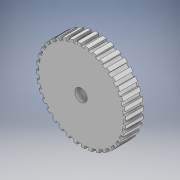
# Autodesk Inventor part: IPC BRT Knob
Saved by Autodesk Inventor 2022 (Build 260153000, 153)
## iProperties
Created: 2022-01-01
Part Number: IPC BRT Knob
Material: Generic
Document SubType Name: Modeling
Designer: solor
Density: 1 g/cm^3
Appearance: Default
Author: solor
Autodesk Inventor part; units mm, degrees
ref_plane "YZ Plane" through (0, 0, 0) normal (1, 0, 0) x (0, 1, 0)
ref_plane "XZ Plane" through (0, 0, 0) normal (0, 1, 0) x (-1, 0, 0)
sketch "Sketch1" plane through (0, 0, 0) normal (0, 0, 1) x (1, 0, 0)
  arc A0 (21.6935, 0) -> (21.6109, 1.8907) centre (0, 0) ccw
  arc A1 (20.422, 1.7867) -> (20.1886, 3.5598) centre (0, 0) ccw
  line L0 (20.422, 1.7867) -> (21.6109, 1.8907)
  line L1 (20.1886, 3.5598) -> (21.3639, 3.767)
  arc A2 (21.3639, 3.767) -> (20.9543, 5.6147) centre (0, 0) ccw
  arc A3 (19.8015, 5.3058) -> (19.2637, 7.0114) centre (0, 0) ccw
  line L2 (19.8015, 5.3058) -> (20.9543, 5.6147)
  line L3 (19.2637, 7.0114) -> (20.3852, 7.4196)
  arc A4 (20.3852, 7.4196) -> (19.661, 9.1681) centre (0, 0) ccw
  arc A5 (18.5793, 8.6637) -> (17.7535, 10.25) centre (0, 0) ccw
  line L4 (18.5793, 8.6637) -> (19.661, 9.1681)
  line L5 (17.7535, 10.25) -> (18.7871, 10.8468)
  arc A6 (18.7871, 10.8467) -> (17.7703, 12.4429) centre (0, 0) ccw
  arc A7 (16.7926, 11.7583) -> (15.7039, 13.1771) centre (0, 0) ccw
  line L6 (16.7926, 11.7583) -> (17.7703, 12.4429)
  line L7 (15.7039, 13.1771) -> (16.6182, 13.9443)
  arc A8 (16.6182, 13.9443) -> (15.3396, 15.3396) centre (0, 0) ccw
  arc A9 (14.4957, 14.4957) -> (13.1771, 15.7039) centre (0, 0) ccw
  line L8 (14.4957, 14.4957) -> (15.3396, 15.3396)
  line L9 (13.1771, 15.7039) -> (13.9443, 16.6182)
  arc A10 (13.9443, 16.6182) -> (12.4429, 17.7703) centre (0, 0) ccw
  arc A11 (11.7583, 16.7926) -> (10.25, 17.7535) centre (0, 0) ccw
  line L10 (11.7583, 16.7926) -> (12.4429, 17.7703)
  line L11 (10.25, 17.7535) -> (10.8468, 18.7871)
  arc A12 (10.8468, 18.7871) -> (9.1681, 19.661) centre (0, 0) ccw
  arc A13 (8.6637, 18.5793) -> (7.0114, 19.2637) centre (0, 0) ccw
  line L12 (8.6637, 18.5793) -> (9.1681, 19.661)
  line L13 (7.0114, 19.2637) -> (7.4196, 20.3852)
  arc A14 (7.4196, 20.3852) -> (5.6147, 20.9543) centre (0, 0) ccw
  arc A15 (5.3058, 19.8015) -> (3.5598, 20.1886) centre (0, 0) ccw
  line L14 (5.3058, 19.8015) -> (5.6147, 20.9543)
  line L15 (3.5598, 20.1886) -> (3.767, 21.3639)
  arc A16 (3.767, 21.3639) -> (1.8907, 21.6109) centre (0, 0) ccw
  arc A17 (1.7867, 20.422) -> (0, 20.5) centre (0, 0) ccw
  line L16 (1.7867, 20.422) -> (1.8907, 21.6109)
  line L17 (0, 20.5) -> (0, 21.6935)
  arc A18 (0, 21.6935) -> (-1.8907, 21.6109) centre (0, 0) ccw
  arc A19 (-1.7867, 20.422) -> (-3.5598, 20.1886) centre (0, 0) ccw
  line L18 (-1.7867, 20.422) -> (-1.8907, 21.6109)
  line L19 (-3.5598, 20.1886) -> (-3.767, 21.3639)
  arc A20 (-3.767, 21.3639) -> (-5.6147, 20.9543) centre (0, 0) ccw
  arc A21 (-5.3058, 19.8015) -> (-7.0114, 19.2637) centre (0, 0) ccw
  line L20 (-5.3058, 19.8015) -> (-5.6147, 20.9543)
  line L21 (-7.0114, 19.2637) -> (-7.4196, 20.3852)
  arc A22 (-7.4196, 20.3852) -> (-9.1681, 19.661) centre (0, 0) ccw
  arc A23 (-8.6637, 18.5793) -> (-10.25, 17.7535) centre (0, 0) ccw
  line L22 (-8.6637, 18.5793) -> (-9.1681, 19.661)
  line L23 (-10.25, 17.7535) -> (-10.8468, 18.7871)
  arc A24 (-10.8467, 18.7871) -> (-12.4429, 17.7703) centre (0, 0) ccw
  arc A25 (-11.7583, 16.7926) -> (-13.1771, 15.7039) centre (0, 0) ccw
  line L24 (-11.7583, 16.7926) -> (-12.4429, 17.7703)
  line L25 (-13.1771, 15.7039) -> (-13.9443, 16.6182)
  arc A26 (-13.9443, 16.6182) -> (-15.3396, 15.3396) centre (0, 0) ccw
  arc A27 (-14.4957, 14.4957) -> (-15.7039, 13.1771) centre (0, 0) ccw
  line L26 (-14.4957, 14.4957) -> (-15.3396, 15.3396)
  line L27 (-15.7039, 13.1771) -> (-16.6182, 13.9443)
  arc A28 (-16.6182, 13.9443) -> (-17.7703, 12.4429) centre (0, 0) ccw
  arc A29 (-16.7926, 11.7583) -> (-17.7535, 10.25) centre (0, 0) ccw
  line L28 (-16.7926, 11.7583) -> (-17.7703, 12.4429)
  line L29 (-17.7535, 10.25) -> (-18.7871, 10.8468)
  arc A30 (-18.7871, 10.8467) -> (-19.661, 9.1681) centre (0, 0) ccw
  arc A31 (-18.5793, 8.6637) -> (-19.2637, 7.0114) centre (0, 0) ccw
  line L30 (-18.5793, 8.6637) -> (-19.661, 9.1681)
  line L31 (-19.2637, 7.0114) -> (-20.3852, 7.4196)
  arc A32 (-20.3852, 7.4196) -> (-20.9543, 5.6147) centre (0, 0) ccw
  arc A33 (-19.8015, 5.3058) -> (-20.1886, 3.5598) centre (0, 0) ccw
  line L32 (-19.8015, 5.3058) -> (-20.9543, 5.6147)
  line L33 (-20.1886, 3.5598) -> (-21.3639, 3.767)
  arc A34 (-21.3639, 3.767) -> (-21.6109, 1.8907) centre (0, 0) ccw
  arc A35 (-20.422, 1.7867) -> (-20.5, 0) centre (0, 0) ccw
  line L34 (-20.422, 1.7867) -> (-21.6109, 1.8907)
  line L35 (-20.5, 0) -> (-21.6935, 0)
  arc A36 (-21.6935, 0) -> (-21.6109, -1.8907) centre (0, 0) ccw
  arc A37 (-20.422, -1.7867) -> (-20.1886, -3.5598) centre (0, 0) ccw
  line L36 (-20.422, -1.7867) -> (-21.6109, -1.8907)
  line L37 (-20.1886, -3.5598) -> (-21.3639, -3.767)
  arc A38 (-21.3639, -3.767) -> (-20.9543, -5.6147) centre (0, 0) ccw
  arc A39 (-19.8015, -5.3058) -> (-19.2637, -7.0114) centre (0, 0) ccw
  line L38 (-19.8015, -5.3058) -> (-20.9543, -5.6147)
  line L39 (-19.2637, -7.0114) -> (-20.3852, -7.4196)
  arc A40 (-20.3852, -7.4196) -> (-19.661, -9.1681) centre (0, 0) ccw
  arc A41 (-18.5793, -8.6637) -> (-17.7535, -10.25) centre (0, 0) ccw
  line L40 (-18.5793, -8.6637) -> (-19.661, -9.1681)
  line L41 (-17.7535, -10.25) -> (-18.7871, -10.8467)
  arc A42 (-18.7871, -10.8467) -> (-17.7703, -12.4429) centre (0, 0) ccw
  arc A43 (-16.7926, -11.7583) -> (-15.7039, -13.1771) centre (0, 0) ccw
  line L42 (-16.7926, -11.7583) -> (-17.7703, -12.4429)
  line L43 (-15.7039, -13.1771) -> (-16.6182, -13.9443)
  arc A44 (-16.6182, -13.9443) -> (-15.3396, -15.3396) centre (0, 0) ccw
  arc A45 (-14.4957, -14.4957) -> (-13.1771, -15.7039) centre (0, 0) ccw
  line L44 (-14.4957, -14.4957) -> (-15.3396, -15.3396)
  line L45 (-13.1771, -15.7039) -> (-13.9443, -16.6182)
  arc A46 (-13.9443, -16.6182) -> (-12.4429, -17.7703) centre (0, 0) ccw
  arc A47 (-11.7583, -16.7926) -> (-10.25, -17.7535) centre (0, 0) ccw
  line L46 (-11.7583, -16.7926) -> (-12.4429, -17.7703)
  line L47 (-10.25, -17.7535) -> (-10.8468, -18.7871)
  arc A48 (-10.8468, -18.7871) -> (-9.1681, -19.661) centre (0, 0) ccw
  arc A49 (-8.6637, -18.5793) -> (-7.0114, -19.2637) centre (0, 0) ccw
  line L48 (-8.6637, -18.5793) -> (-9.1681, -19.661)
  line L49 (-7.0114, -19.2637) -> (-7.4196, -20.3852)
  arc A50 (-7.4196, -20.3852) -> (-5.6147, -20.9543) centre (0, 0) ccw
  arc A51 (-5.3058, -19.8015) -> (-3.5598, -20.1886) centre (0, 0) ccw
  line L50 (-5.3058, -19.8015) -> (-5.6147, -20.9543)
  line L51 (-3.5598, -20.1886) -> (-3.767, -21.3639)
  arc A52 (-3.767, -21.3639) -> (-1.8907, -21.6109) centre (0, 0) ccw
  arc A53 (-1.7867, -20.422) -> (0, -20.5) centre (0, 0) ccw
  line L52 (-1.7867, -20.422) -> (-1.8907, -21.6109)
  line L53 (0, -20.5) -> (0, -21.6935)
  arc A54 (0, -21.6935) -> (1.8907, -21.6109) centre (0, 0) ccw
  arc A55 (1.7867, -20.422) -> (3.5598, -20.1886) centre (0, 0) ccw
  line L54 (1.7867, -20.422) -> (1.8907, -21.6109)
  line L55 (3.5598, -20.1886) -> (3.767, -21.3639)
  arc A56 (3.767, -21.3639) -> (5.6147, -20.9543) centre (0, 0) ccw
  arc A57 (5.3058, -19.8015) -> (7.0114, -19.2637) centre (0, 0) ccw
  line L56 (5.3058, -19.8015) -> (5.6147, -20.9543)
  line L57 (7.0114, -19.2637) -> (7.4196, -20.3852)
  arc A58 (7.4196, -20.3852) -> (9.1681, -19.661) centre (0, 0) ccw
  arc A59 (8.6637, -18.5793) -> (10.25, -17.7535) centre (0, 0) ccw
  line L58 (8.6637, -18.5793) -> (9.1681, -19.661)
  line L59 (10.25, -17.7535) -> (10.8467, -18.7871)
  arc A60 (10.8468, -18.7871) -> (12.4429, -17.7703) centre (0, 0) ccw
  arc A61 (11.7583, -16.7926) -> (13.1771, -15.7039) centre (0, 0) ccw
  line L60 (11.7583, -16.7926) -> (12.4429, -17.7703)
  line L61 (13.1771, -15.7039) -> (13.9443, -16.6182)
  arc A62 (13.9443, -16.6182) -> (15.3396, -15.3396) centre (0, 0) ccw
  arc A63 (14.4957, -14.4957) -> (15.7039, -13.1771) centre (0, 0) ccw
  line L62 (14.4957, -14.4957) -> (15.3396, -15.3396)
  line L63 (15.7039, -13.1771) -> (16.6182, -13.9443)
  arc A64 (16.6182, -13.9443) -> (17.7703, -12.4429) centre (0, 0) ccw
  arc A65 (16.7926, -11.7583) -> (17.7535, -10.25) centre (0, 0) ccw
  line L64 (16.7926, -11.7583) -> (17.7703, -12.4429)
  line L65 (17.7535, -10.25) -> (18.7871, -10.8468)
  arc A66 (18.7871, -10.8468) -> (19.661, -9.1681) centre (0, 0) ccw
  arc A67 (18.5793, -8.6637) -> (19.2637, -7.0114) centre (0, 0) ccw
  line L66 (18.5793, -8.6637) -> (19.661, -9.1681)
  line L67 (19.2637, -7.0114) -> (20.3852, -7.4196)
  arc A68 (20.3852, -7.4196) -> (20.9543, -5.6147) centre (0, 0) ccw
  arc A69 (19.8015, -5.3058) -> (20.1886, -3.5598) centre (0, 0) ccw
  line L68 (19.8015, -5.3058) -> (20.9543, -5.6147)
  line L69 (20.1886, -3.5598) -> (21.3639, -3.767)
  arc A70 (21.3639, -3.767) -> (21.6109, -1.8907) centre (0, 0) ccw
  arc A71 (20.422, -1.7867) -> (20.5, 0) centre (0, 0) ccw
  line L70 (20.422, -1.7867) -> (21.6109, -1.8907)
  line L71 (20.5, 0) -> (21.6935, 0)
  dimension "d7" = 360
  constraints: 180 point on circle, 144 end point, 72 centre point, 37 coincident, 397 other
extrude "Extrusion1" add sketch "Sketch1" along normal blind 8.6
sketch "Sketch2" plane through (0, 0, 8.6) normal (0, 0, 1) x (1, 0, 0)
  circle A0 centre (0, 0) radius 2.9
  dimension "d11" = 5.8
  constraints: 1 centre point, 1 coincident
  measures "d11" diameter of A0
extrude "Extrusion2" cut sketch "Sketch2" against normal blind 9.8875
sketch "Sketch3" plane through (0, 0, 8.6) normal (0, 0, 1) x (1, 0, 0)
  circle A0 centre (0, 0) radius 3.5
  dimension "d14" = 7
  constraints: 1 centre point, 1 coincident
  measures "d14" diameter of A0
sketch "Sketch4" plane through (0, 0, 8.6) normal (0, 0, 1) x (1, 0, 0)
  circle A0 centre (0, 0) radius 2.9
  circle A1 centre (0, 0) radius 5.25
  dimension "d17" = 10.5
  constraints: 2 centre point, 2 coincident
  measures "d17" diameter of A1
ref_plane "Work Plane1" through (0, 0, 9.6) normal (0, 0, 1) x (1, 0, 0)
sketch "Sketch5" plane through (0, 0, 9.6) normal (0, 0, 1) x (1, 0, 0)
  circle A0 centre (0, 0) radius 2.9 projected
  circle A1 centre (0, 0) radius 2.96
  dimension "d22" = 0.06
  dimension "d23" = 5.8
  constraints: 1 centre point
  measures "d22" radial gap between concentric circles of A0 A1
  measures "d23" diameter of A0
extrude "Extrusion5" cut sketch "Sketch5" against normal blind 9.3 contours A0 | A1
sketch "Sketch6" plane through (0, 0, 8.6) normal (0, 0, 1) x (1, 0, 0)
  circle A0 centre (0, 0) radius 2.96 projected
  circle A1 centre (0, 0) radius 6.0945
  constraints: 1 centre point, 1 coincident
sketch "Sketch7" plane through (0, 0, 0) normal (1, 0, 0) x (0, 1, 0)
  line L0 (2.96, 6.9) -> (-2.96, 6.9) projected
  line L1 (-2.96, 0.3) -> (2.96, 0.3) projected
  point P0 (0, 0)
  dimension "d30" = 6.6
  measures "d30" distance between parallel lines of L1 L0
body "Solid1"
